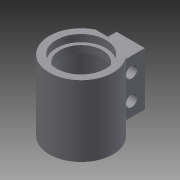
# Autodesk Inventor part: brush holder v4
Saved by Autodesk Inventor 2013 SP2 (Build 170200200, 200)
## iProperties
Created: 2017-05-15
Part Number: brush holder v4
Material: Generic
Document SubType Name: Modeling
Designer: Herman de Vries
Density: 1 g/cm^3
Author: Herman de Vries
Autodesk Inventor part; units mm, degrees
ref_plane "YZ Plane" through (0, 0, 0) normal (1, 0, 0) x (0, 1, 0)
ref_plane "XZ Plane" through (0, 0, 0) normal (0, 1, 0) x (-1, 0, 0)
ref_plane "XY Plane" through (0, 0, 0) normal (0, 0, 1) x (1, 0, 0)
sketch "Sketch1" plane through (0, 0, 0) normal (1, 0, 0) x (0, 1, 0)
  line L0 (0, 18) -> (5.825, 18) construction
  line L1 (0, 0) -> (7.3998, 0) construction
  line L2 (0, 12.5) -> (0, 0) construction
  line L3 (7.3998, 0) -> (9, 0) construction
  line L4 (9, 0) -> (9, 18)
  line L5 (9, 18) -> (9, 18)
  line L6 (9, 18) -> (9, 20)
  line L7 (9, 20) -> (7, 20)
  line L8 (7, 20) -> (7, 18)
  line L9 (5.825, 18) -> (7, 18) construction
  line L10 (5.825, 18) -> (7.3998, 0) construction
  line L11 (6, 18) -> (7, 18)
  line L12 (6, 16) -> (7.3998, 0)
  line L13 (9, 0) -> (7.3998, 0)
  line L14 (6, 18) -> (6, 16)
  point P0 (2.25, 0)
  dimension "d2" = 18
  dimension "d12" = 2
  dimension "d14" = 0
  dimension "d16" = 2
  dimension "d17" = 7
  dimension "d35" = 95
  dimension "d36" = 9
  dimension "d57" = 2
  dimension "d60" = 6
  constraints: 30 end point, 5 parallel, 3 collinear, 3 perpendicular, 3 point on line, 1 horizontal, 1 vertical, 1 vertical alignment
  measures "d2" distance between parallel lines of L0 L1
  measures "d12" distance of L5.end L6.end
  measures "d14" distance of L4.end L5.end
  measures "d16" distance of L8.end L7.end
  measures "d17" distance between parallel lines of L2 L8
  measures "d35" angle of L10 L3
  measures "d36" distance from line of L4 L1.start
  measures "d57" distance of L12.start L11.start
  measures "d60" distance between parallel lines of L2 L14
revolve "Revolution1" add sketch "Sketch1" angle 360 about axis through (0, 0, 12.5) along (0, 0, -1)
sketch "Sketch3" plane through (0, 0, 0) normal (1, 0, 0) x (0, 1, 0)
  line L0 (14, 0) -> (14, 18)
  line L1 (14, 18) -> (7.3998, 18)
  line L2 (14, 0) -> (7.3998, 0)
  line L3 (-7.3998, 0) -> (7.3998, 0) projected
  line L4 (7.3998, 0) -> (7.3998, 18)
  line L5 (-6, 18) -> (6, 18) projected
  point P0 (0, 0)
  dimension "d28" = 14
  constraints: 8 end point, 1 collinear, 1 vertical
  measures "d28" distance from line of L0 point (0, 0)
extrude "Extrusion1" add sketch "Sketch3" along normal mid plane 8
sketch "Sketch4" plane through (-4, 0, 0) normal (-1, 0, 0) x (0, 0, 1)
  circle A0 centre (5.5, 10.25) radius 1.6
  circle A1 centre (12.5, 10.25) radius 1.6
  line L0 (5.5, 10.25) -> (12.5, 10.25) construction
  line L1 (18, 14) -> (0, 14) construction
  point P0 (0, 0)
  point P1 (17, 10.25)
  point P2 (9, 10.25)
  point P3 (9, 14)
  dimension "d29" = 3.2
  dimension "d30" = 3.2
  dimension "d31" = 7
  dimension "d34" = 3.75
  constraints: 2 centre point, 2 end point, 2 horizontal alignment, 2 midpoint, 1 horizontal, 1 vertical alignment
  measures "d29" diameter of A0
  measures "d30" diameter of A1
  measures "d31" distance of L0.start L0.end
  measures "d34" distance between parallel lines of L0 L1
extrude "Extrusion2" cut sketch "Sketch4" against normal blind 10
sketch "Sketch5" plane through (4, 0, 0) normal (1, 0, 0) x (0, 0, -1)
  circle A0 centre (-5.5, 10.25) radius 1.6 projected
  circle A1 centre (-12.5, 10.25) radius 1.6 projected
  line L0 (0, 8.0623) -> (-18, 8.0623) projected
  line L1 (-20.496, 14) -> (-16.5, 14)
  line L2 (-16.5, 14) -> (-16.5, 8.0623)
  line L3 (-16.5, 8.0623) -> (-20.496, 8.0623)
  line L4 (-20.496, 8.0623) -> (-20.496, 14)
  line L5 (0, 14) -> (-1.5, 14)
  line L6 (-1.5, 14) -> (-1.5, 8.0623)
  line L7 (-1.5, 8.0623) -> (0, 8.0623)
  line L8 (0, 8.0623) -> (0, 14)
  line L9 (0, 14) -> (-18, 14) projected
  point P0 (0, 0)
  dimension "d47" = 15
  dimension "d49" = 4
  dimension "d50" = 4
  constraints: 16 end point, 4 parallel, 2 horizontal, 2 perpendicular, 2 point on line, 1 collinear
  measures "d47" distance between parallel lines of L6 L2
  measures "d49" distance from line of L2 A1.centre
  measures "d50" distance from line of L6 A0.centre
extrude "Extrusion3" cut sketch "Sketch5" against normal blind 10 contours L0 L6 L5 L8 | L0 L3 L4 L1 L2
equation "\"d49\" = d50"
body "Solid1"
